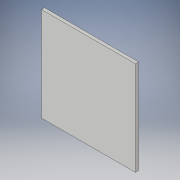
# Autodesk Inventor part: PythonKukaFloor
Saved by Autodesk Inventor 2019.1 (Build 231200000, 200)
## iProperties
Created: 2020-09-13
Part Number: PythonKukaFloor
Material: Generic
Document SubType Name: Modeling
Designer: lucas
Density: 1 g/cm^3
Appearance: Default
Author: lucas
Autodesk Inventor part; units mm, degrees
ref_plane "YZ Plane" through (0, 0, 0) normal (1, 0, 0) x (0, 1, 0)
ref_plane "XZ Plane" through (0, 0, 0) normal (0, 1, 0) x (-1, 0, 0)
ref_plane "XY Plane" through (0, 0, 0) normal (0, 0, 1) x (1, 0, 0)
sketch "Sketch1" plane through (0, 0, 0) normal (0, 0, 1) x (1, 0, 0)
  line L0 (-300, 300) -> (300, 300)
  line L1 (300, 300) -> (300, -300)
  line L2 (300, -300) -> (-300, -300)
  line L3 (-300, -300) -> (-300, 300)
  point P0 (0, 0)
  dimension "d0" = 600
  dimension "d1" = 600
  dimension "d2" = 300
  dimension "d3" = 300
  constraints: 8 end point, 2 parallel, 1 horizontal, 1 perpendicular
  measures "d0" distance of L0.start L0.end
  measures "d1" distance of L2.end L0.start
  measures "d2" distance from line of point (0, 0) L0
  measures "d3" distance from line of point (0, 0) L3
extrude "Extrusion1" add sketch "Sketch1" along normal blind 20
equation "\"d1\" = d0"
equation "\"d2\" = 0.5 * d1"
equation "\"d3\" = 0.5 * d0"
body "Solid1"
